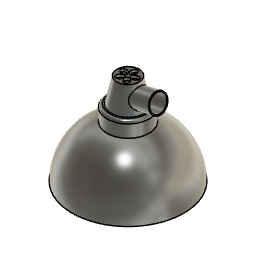
Q1 (Autodesk Fusion 360 archive; units mm, degrees)
design "HOLDER"
Autodesk Fusion 360 part; units mm, degrees
note: some values were not read from the file. Chosen so that the rebuilt part matches the saved one: where a step ends.
sketch "Sketch1" plane through (0, 0, 0) normal (0, 1, 0) x (1, 0, 0)
  line L0 (0, -100) -> (0, 0)
  line L1 (0, 0) -> (100, 0)
  arc A0 (0, -100) -> (100, 0) centre (0, 0) ccw
  dimension "d1" = 200
  constraint coincident L0.end L1.start
  constraint vertical L0
  constraint perpendicular L0 L1
  measures "d1" diameter of A0
revolve "Revolve1" add sketch "Sketch1" angle 360 about axis through (0, 0, 100) along (0, 0, -1)
shell "Shell1" thickness 2 removed faces 1 at (-27.5413, -26.5675, 0)
sketch "Sketch2" plane through (0, 0, 0) normal (0, 1, 0) x (1, 0, 0)
ref_plane "WorkPlane1" through (0, 0, 100) normal (0, 0, 1) x (1, 0, 0)
sketch "Sketch3" plane through (0, 0, 100) normal (0, 0, 1) x (1, 0, 0)
  circle A0 centre (0, 0) radius 37.5
  dimension "d5" = 75
  constraint coincident A0.centre origin
  measures "d5" diameter of A0
extrude "Extrude1" add sketch "Sketch3" along normal up to surface end surface at (49.5722, 85.8616, 13.0526)
extrude "Extrude2" add 1 faces at (9.3028, 10.3652, 100) along direction (0, 0, 1) blind 20
fillet "Fillet1" radius 5 1 edges at (-34.9623, -13.5606, 120)
sketch "Sketch4" plane through (0, 0, 120) normal (0, 0, 1) x (-1, 0, 0)
  circle A0 centre (0, 0) radius 32.5
sketch "Sketch5" plane through (0, 0, 0) normal (1, 0, 0) x (0, 1, 0)
  line L0 (0, 120) -> (0, 163.5901)
  line L1 (0, 163.5901) -> (-20, 163.5901)
  line L2 (-20, 163.5901) -> (-30, 120)
  line L3 (-30, 120) -> (0, 120)
  line L4 (0, 180) -> (0, 104.7628) construction
  constraint vertical L0
  constraint perpendicular L0 L1
  constraint perpendicular L0 L3
  constraint vertical L4
revolve "Revolve2" add sketch "Sketch5" angle 360 about axis through (0, 0, 180) along (0, 0, -1)
ref_plane "WorkPlane2" through (25, 0, 141.7951) normal (0.974681, 0, 0.223601) x (0, -1, 0)
sketch "Sketch6" plane through (25, 0, 141.7951) normal (0.974681, 0, 0.223601) x (0, -1, 0)
  circle A0 centre (0.2894, 0.5098) radius 17
  circle A1 centre (0.2894, 0.5098) radius 15
  dimension "d14" = 34
  dimension "d15" = 30
  constraint concentric A0 A1
  measures "d14" diameter of A0
  measures "d15" diameter of A1
extrude "Extrude3" add sketch "Sketch6" along normal up to near side of body 1
extrude "Extrude4" add 1 faces at (21.4794, 0.8343, 157.1413) along direction (0.974681, 0, 0.223601) blind 30
sketch "Sketch7" plane through (0, 0, 163.5901) normal (0, 0, 1) x (-1, 0, 0)
  circle A0 centre (0, 0) radius 20
  ellipse E0 centre (0.2213, -10.3311) end of major axis (0.2213, -17.1293) minor radius 5.0076
  line L0 (0.2213, -3.533) -> (0.2213, -17.1293)
  line L1 (-4.7863, -10.3311) -> (5.229, -10.3311)
  ellipse E1 centre (9.8939, -2.982) end of major axis (16.3593, -5.0827) minor radius 5.0076
  ellipse E2 centre (5.8934, 8.4882) end of major axis (9.8893, 13.988) minor radius 5.0076
  ellipse E3 centre (-6.2515, 8.2279) end of major axis (-10.2474, 13.7278) minor radius 5.0076
  ellipse E4 centre (-9.7571, -3.403) end of major axis (-16.2225, -5.5037) minor radius 5.0076
  dimension "d21" = 360
  constraint vertical L0
  constraint coincident E0 L0.start
  constraint coincident E0 L0.end
  constraint coincident E0 L1.start
  constraint coincident E0 L1.end
extrude "Extrude5" cut sketch "Sketch7" against normal blind 5 contours E0 L0 L1 | E0 L0 L1 | E0 L0 L1 | E0 L0 L1 | E1 | E2 | E3 | E4
